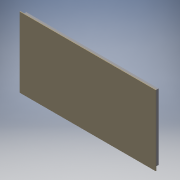
# Autodesk Inventor part: gatorboard_01875in_front_door
Saved by Autodesk Inventor 2019 (Build 230136000, 136)
## iProperties
Created: 2019-03-10
Part Number: gatorboard_01875in_front_door
Material: Generic
Document SubType Name: Modeling
Designer: Wilson Lab
Density: 1 g/cm^3
Appearance: Default
Author: Wilson Lab
Autodesk Inventor part; units mm, degrees
ref_plane "YZ Plane" through (0, 0, 0) normal (1, 0, 0) x (0, 1, 0)
ref_plane "XZ Plane" through (0, 0, 0) normal (0, 1, 0) x (-1, 0, 0)
ref_plane "XY Plane" through (0, 0, 0) normal (0, 0, 1) x (1, 0, 0)
sketch "Sketch1" plane through (0, 0, 0) normal (0, 0, 1) x (1, 0, 0)
  line L0 (0, 0) -> (861.06, 0)
  line L1 (861.06, 0) -> (861.06, 444.5)
  line L2 (861.06, 444.5) -> (0, 444.5)
  line L3 (0, 444.5) -> (0, 0)
  dimension "d2" = 861.06
  dimension "d3" = 444.5
  constraints: 8 end point, 2 parallel, 1 coincident, 1 horizontal, 1 perpendicular
  measures "d2" distance of L1.end L2.end
  measures "d3" distance of L0.end L1.end
extrude "Extrusion1" add sketch "Sketch1" along normal blind 4.7625
sketch "Sketch2" plane through (0, 0, 0) normal (0, 0, -1) x (-1, 0, 0)
  line L0 (-11.43, 13.2197) -> (-11.43, 470.4197) projected
  line L1 (-849.63, 432.3197) -> (-11.43, 432.3197) projected
  line L2 (-887.73, 13.2197) -> (26.67, 13.2197) projected
  line L3 (-849.63, 470.4197) -> (-849.63, 13.2197) projected
  line L4 (-849.63, 13.2197) -> (-11.43, 13.2197)
  line L5 (-11.43, 13.2197) -> (-11.43, 432.3197)
  line L6 (-11.43, 432.3197) -> (-849.63, 432.3197)
  line L7 (-849.63, 432.3197) -> (-849.63, 13.2197)
  point P0 (0, 0)
  constraints: 8 end point, 2 parallel, 1 horizontal, 1 perpendicular
extrude "Extrusion2" add sketch "Sketch2" along normal blind 25.4
body "Solid1"
